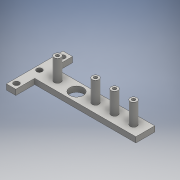
# Autodesk Inventor part: Kroller Holder
Saved by Autodesk Inventor 2016 (Build 200138000, 138)
## iProperties
Created: 2018-03-02
Part Number: Kroller Holder
Material: Generic
Document SubType Name: Modeling
Designer: Simon
Density: 1 g/cm^3
Appearance: Default
Author: Simon
Autodesk Inventor part; units mm, degrees
ref_plane "YZ Plane" through (0, 0, 0) normal (1, 0, 0) x (0, 1, 0)
ref_plane "XZ Plane" through (0, 0, 0) normal (0, 1, 0) x (-1, 0, 0)
ref_plane "XY Plane" through (0, 0, 0) normal (0, 0, 1) x (1, 0, 0)
sketch "Sketch1" plane through (0, 0, 0) normal (0, 0, 1) x (1, 0, 0)
  line L0 (0, 0) -> (42, 0)
  line L1 (42, 0) -> (42, 14)
  line L2 (42, 14) -> (0, 14)
  line L3 (0, 14) -> (0, 0)
  dimension "d0" = 42
  dimension "d1" = 14
  constraints: 8 end point, 2 parallel, 1 horizontal, 1 perpendicular
  measures "d0" distance of L2.end L1.end
  measures "d1" distance of L1.end L0.end
extrude "Extrusion1" add sketch "Sketch1" along normal blind 4
sketch "Sketch2" plane through (0, 0, 4) normal (0, 0, 1) x (1, 0, 0)
  circle A0 centre (21, 7) radius 2.55
  line L0 (42, 14) -> (0, 14) projected
  line L1 (0, 14) -> (0, 0) projected
  circle A1 centre (6.9, 7) radius 2.5
  circle A2 centre (35.1, 7) radius 2.5
  dimension "d35" = 0
  dimension "d4" = 5.1
  dimension "d5" = 42
  dimension "d6" = 14
  dimension "d7" = 7
  dimension "d8" = 21
  dimension "d9" = 5
  dimension "d10" = 5
  dimension "d11" = 14.1
  dimension "d12" = 14.1
  constraints: 3 centre point
  measures "d4" diameter of A0
  measures "d5" distance of L0.start L0.end
  measures "d6" distance of L0.end L1.end
  measures "d7" distance from line of L0 A0.centre
  measures "d8" distance from line of L1 A0.centre
  measures "d9" diameter of A1
  measures "d10" diameter of A2
  measures "d11" distance of A0.centre A1.centre
  measures "d12" distance of A2.centre A0.centre
extrude "Extrusion2" add sketch "Sketch2" along normal blind 16 contours A1 | A2
extrude "Extrusion3" cut sketch "Sketch2" against normal blind 4 contours A0
sketch "Sketch3" plane through (6.9, 7, 20) normal (0, 0, 1) x (1, 0, 0)
  circle A0 centre (0, 0) radius 1.25
  circle A1 centre (28.2, 0) radius 2.5 projected
  circle A2 centre (28.2, 0) radius 1.25
  point P0 (-6.9, -7)
  dimension "d19" = 2.5
  dimension "d20" = 2.5
  constraints: 2 centre point, 1 coincident
  measures "d19" diameter of A0
  measures "d20" diameter of A2
extrude "Extrusion4" cut sketch "Sketch3" against normal blind 3 contours A0 | A2
sketch "Sketch4" plane through (0, 0, 0) normal (0, 0, -1) x (-1, 0, 0)
  circle A0 centre (-21, 7) radius 2.55 projected
  circle A1 centre (-49.8, 7) radius 2.55
  point P0 (0, 0)
  dimension "d23" = 5.1
  dimension "d24" = 28.8
  constraints: 1 centre point
  measures "d23" diameter of A1
  measures "d24" distance of A1.centre A0.centre
sketch "Sketch5" plane through (42, 0, 0) normal (1, 0, 0) x (0, 0, -1)
  line L0 (0, 0) -> (-4, 0) projected
  line L1 (-4, 14) -> (0, 14)
  line L2 (0, 14) -> (0, 0)
  line L3 (0, 0) -> (-4, 0)
  line L4 (-4, 0) -> (-4, 14)
  constraints: 8 end point, 2 parallel, 1 horizontal, 1 perpendicular
extrude "Extrusion5" add sketch "Sketch5" along normal blind 30
extrude "Extrusion6" cut sketch "Sketch4" against normal blind 2 contours A1
sketch "Sketch6" plane through (0, 0, 0) normal (0, 0, -1) x (-1, 0, 0)
  circle A0 centre (-21, 7) radius 2.55 projected
  circle A1 centre (-21, 7) radius 5.05
  point P0 (0, 0)
  dimension "d29" = 10.1
  constraints: 1 centre point, 1 coincident
  measures "d29" diameter of A1
extrude "Extrusion7" cut sketch "Sketch6" against normal through all
sketch "Sketch7" plane through (0, 0, 4) normal (0, 0, 1) x (1, 0, 0)
  circle A0 centre (35.1, 7) radius 2.5 projected
  circle A1 centre (49.2, 7) radius 2.5
  point P0 (0, 0)
  dimension "d32" = 5
  dimension "d33" = 14.1
  constraints: 1 centre point
  measures "d32" diameter of A1
  measures "d33" distance of A0.centre A1.centre
extrude "Extrusion8" add sketch "Sketch7" along normal blind 16 contours A1
fillet "Fillet3" radius 1 1 edges at (52.35, 7, 2)
sketch "Sketch8" plane through (49.2, 7, 20) normal (0, 0, 1) x (1, 0, 0)
  circle A0 centre (0, 0) radius 1.25
  point P0 (-49.2, -7)
  dimension "d37" = 2.5
  constraints: 1 centre point
  measures "d37" diameter of A0
extrude "Extrusion9" cut sketch "Sketch8" against normal blind 3
pattern_linear "Rectangular Pattern1" count 2 spacing 14.1 along (1, 0, 0) of "Extrusion8", "Extrusion9"
sketch "Sketch9" plane through (0, 0, 0) normal (-1, 0, 0) x (0, 0, 1)
  line L0 (4, 14) -> (4, 0) projected
  line L1 (0, 0) -> (4, 0)
  line L2 (4, 0) -> (4, 14)
  line L3 (4, 14) -> (0, 14)
  line L4 (0, 14) -> (0, 0)
  constraints: 8 end point, 2 parallel, 1 horizontal, 1 perpendicular
extrude "Extrusion10" add sketch "Sketch9" along normal blind 10
sketch "Sketch10" plane through (72, 0, 0) normal (0, -1, 0) x (1, 0, 0)
  line L0 (0, 4) -> (-82, 4) projected
  line L1 (-82, 0) -> (0, 0) projected
  line L2 (-82, 4) -> (-75, 4)
  line L3 (-75, 4) -> (-75, 0)
  line L4 (-75, 0) -> (-82, 0)
  line L5 (-82, 0) -> (-82, 4)
  point P0 (-72, 0)
  dimension "d46" = 7
  constraints: 8 end point, 2 parallel, 1 horizontal, 1 perpendicular, 1 point on line
  measures "d46" distance of L3.end L4.end
extrude "Extrusion11" add sketch "Sketch10" along normal blind 14
sketch "Sketch11" plane through (72, 14, 4) normal (0, 1, 0) x (1, 0, 0)
  line L0 (-82, 0) -> (-82, 4) projected
  line L1 (-82, 4) -> (-75, 4) projected
  line L2 (-82, 0) -> (-75, 0)
  line L3 (-75, 0) -> (-75, 4)
  line L4 (-75, 4) -> (-82, 4)
  line L5 (-82, 4) -> (-82, 0)
  point P0 (-72, 4)
  dimension "d49" = 7
  constraints: 8 end point, 2 parallel, 1 horizontal, 1 perpendicular
  measures "d49" distance of L4.end L1.end
extrude "Extrusion12" add sketch "Sketch11" along normal blind 14
sketch "Sketch12" plane through (0, 0, 4) normal (0, 0, 1) x (1, 0, 0)
  circle A0 centre (-6.5, 24) radius 2.05
  line L0 (-3, 14) -> (-3, 28) projected
  line L1 (-10, 28) -> (-3, 28) projected
  circle A1 centre (-6.5, 7) radius 2.05
  circle A2 centre (-6.5, -10) radius 2.05
  point P0 (0, 0)
  dimension "d52" = 4.1
  dimension "d53" = 3.5
  dimension "d54" = 4
  dimension "d57" = 17
  constraints: 3 centre point, 1 vertical, 4 other
  measures "d52" diameter of A0
  measures "d53" distance from line of L0 A0.centre
  measures "d54" distance from line of L1 A0.centre
  measures "d57" distance of A0.centre A1.centre
extrude "Extrusion13" cut sketch "Sketch12" against normal through all
equation "\"d7\" = 0.5 * d6"
equation "\"d8\" = 0.5 * d5"
body "Solid1"
